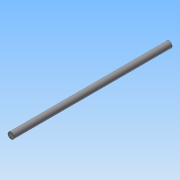
# Autodesk Inventor part: schaft1
Saved by Autodesk Inventor 2015 (Build 190159000, 159)
## iProperties
Created: 2014-08-31
Part Number: schaft1
Material: Generic
Document SubType Name: Modeling
Designer: shohei
Density: 1 g/cm^3
Appearance: Default
Author: shohei
Autodesk Inventor part; units mm, degrees
ref_plane "YZ Plane" through (0, 0, 0) normal (1, 0, 0) x (0, 1, 0)
ref_plane "XZ Plane" through (0, 0, 0) normal (0, 1, 0) x (-1, 0, 0)
ref_plane "XY Plane" through (0, 0, 0) normal (0, 0, 1) x (1, 0, 0)
sketch "Sketch1" plane through (0, 0, 0) normal (0, 1, 0) x (-1, 0, 0)
  circle A0 centre (0, 0) radius 5
  dimension "d0" = 10
  constraints: 1 centre point, 1 coincident
  measures "d0" diameter of A0
extrude "Extrusion1" add sketch "Sketch1" along normal blind 150 and the other way blind 100
sketch "Sketch2" plane through (0, -100, 0) normal (0, -1, 0) x (1, 0, 0)
  point P0 (0, 0)
body "Solid1"
